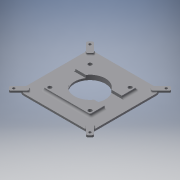
# Autodesk Inventor part: LX4000 Cuvette adapter
Saved by Autodesk Inventor 2016 (Build 200138000, 138)
## iProperties
Created: 2015-05-08
Part Number: LX4000 Cuvette adapter
Material: Generic
Document SubType Name: Modeling
Designer: kthorn
Density: 1 g/cm^3
Appearance: Default
Author: kthorn
Autodesk Inventor part; units mm, degrees
ref_plane "YZ Plane" through (0, 0, 0) normal (1, 0, 0) x (0, 1, 0)
ref_plane "XZ Plane" through (0, 0, 0) normal (0, 1, 0) x (-1, 0, 0)
ref_plane "XY Plane" through (0, 0, 0) normal (0, 0, 1) x (1, 0, 0)
sketch "Sketch1" plane through (0, 0, 0) normal (0, 0, 1) x (1, 0, 0)
  line L0 (-34.939227, 36.850829) -> (65.060773, 36.850829)
  line L1 (73.060773, 28.850829) -> (73.060773, -71.149171)
  line L2 (65.060773, -79.149171) -> (-34.939227, -79.149171)
  line L3 (-42.939227, -71.149171) -> (-42.939227, 28.850829)
  arc A0 (-34.939227, 36.850829) -> (-42.939227, 28.850829) centre (-34.939227, 28.850829) ccw
  arc A1 (-42.939227, -71.149171) -> (-34.939227, -79.149171) centre (-34.939227, -71.149171) ccw
  arc A2 (65.060773, -79.149171) -> (73.060773, -71.149171) centre (65.060773, -71.149171) ccw
  arc A3 (73.060773, 28.850829) -> (65.060773, 36.850829) centre (65.060773, 28.850829) ccw
  point P0 (0, 0)
  point P1 (-42.939227, 36.850829)
  point P2 (73.060773, 36.850829)
  dimension "d0" = 116
  dimension "d2" = 8
  constraints: 8 end point, 8 point on circle, 8 tangent, 4 centre point, 4 point on line, 3 equal radius, 2 parallel, 2 perpendicular, 1 horizontal
  measures "d0" distance of point (-42.939, 36.851) point (73.061, 36.851)
  measures "d2" radius of A0
extrude "Extrusion1" add sketch "Sketch1" along normal blind 3.1
sketch "Sketch3" plane through (0, 0, 3.1) normal (0, 0, 1) x (1, 0, 0)
  line L0 (-34.939227, -79.149171) -> (65.060773, -79.149171)
  line L1 (65.060773, 36.850829) -> (-34.939227, 36.850829)
  line L2 (-42.939227, -71.149171) -> (-42.939227, -79.149171) construction
  line L3 (-34.939227, -79.149171) -> (-42.939227, -79.149171) construction
  line L4 (-42.939227, -79.149171) -> (-42.939227, -82.899171) construction
  line L5 (-42.939227, -82.899171) -> (-46.689227, -82.899171) construction
  line L6 (-32.658004, -75.231909) -> (-46.093032, -88.666938)
  line L7 (-48.92146, -88.666938) -> (-52.456993, -85.131404)
  line L8 (-52.456993, -82.302977) -> (-39.021965, -68.867948)
  line L9 (-36.193538, -68.867948) -> (-32.658004, -72.403482)
  line L10 (-46.689227, -82.899171) -> (-46.689227, -86.899171) construction
  line L11 (-46.689227, -86.899171) -> (-50.689227, -86.899171) construction
  circle A0 centre (-46.689227, -82.899171) radius 2
  arc A1 (-52.456993, -82.302977) -> (-52.456993, -85.131404) centre (-51.04278, -83.71719) ccw
  arc A2 (-48.92146, -88.666938) -> (-46.093032, -88.666938) centre (-47.507246, -87.252724) ccw
  arc A3 (-36.193538, -68.867948) -> (-39.021965, -68.867948) centre (-37.607751, -70.282162) ccw
  arc A4 (-32.658004, -75.231909) -> (-32.658004, -72.403482) centre (-34.072217, -73.817696) ccw
  line L12 (-42.939227, 28.850829) -> (-42.939227, -71.149171)
  arc A5 (-42.939227, -71.149171) -> (-34.939227, -79.149171) centre (-34.939227, -71.149171) ccw
  line L13 (-34.939227, -79.149171) -> (65.060773, -79.149171)
  arc A6 (65.060773, -79.149171) -> (73.060773, -71.149171) centre (65.060773, -71.149171) ccw
  line L14 (73.060773, -71.149171) -> (73.060773, 28.850829)
  arc A7 (73.060773, 28.850829) -> (65.060773, 36.850829) centre (65.060773, 28.850829) ccw
  line L15 (65.060773, 36.850829) -> (-34.939227, 36.850829)
  arc A8 (-34.939227, 36.850829) -> (-42.939227, 28.850829) centre (-34.939227, 28.850829) ccw
  line L16 (15.060773, -79.149171) -> (15.060773, 36.850829) construction
  line L17 (73.060773, -21.149171) -> (-42.939227, -21.149171) construction
  line L18 (73.060773, -71.149171) -> (73.060773, -79.149171) construction
  line L19 (65.060773, -79.149171) -> (73.060773, -79.149171) construction
  line L20 (73.060773, -79.149171) -> (73.060773, -82.899171) construction
  line L21 (73.060773, -82.899171) -> (76.810773, -82.899171) construction
  line L22 (62.779551, -75.231909) -> (76.214579, -88.666938)
  line L23 (79.043007, -88.666938) -> (82.57854, -85.131404)
  line L24 (82.57854, -82.302977) -> (69.143512, -68.867948)
  line L25 (66.315084, -68.867948) -> (62.779551, -72.403482)
  line L26 (76.810773, -82.899171) -> (76.810773, -86.899171) construction
  line L27 (76.810773, -86.899171) -> (80.810773, -86.899171) construction
  circle A9 centre (76.810773, -82.899171) radius 2
  arc A10 (82.57854, -85.131404) -> (82.57854, -82.302977) centre (81.164327, -83.71719) ccw
  arc A11 (76.214579, -88.666938) -> (79.043007, -88.666938) centre (77.628793, -87.252724) ccw
  arc A12 (69.143512, -68.867948) -> (66.315084, -68.867948) centre (67.729298, -70.282162) ccw
  arc A13 (62.779551, -72.403482) -> (62.779551, -75.231909) centre (64.193764, -73.817696) ccw
  arc A14 (65.060773, -79.149171) -> (73.060773, -71.149171) centre (65.060773, -71.149171) ccw
  line L28 (-42.939227, 28.850829) -> (-42.939227, 36.850829) construction
  line L29 (-34.939227, 36.850829) -> (-42.939227, 36.850829) construction
  line L30 (-42.939227, 36.850829) -> (-42.939227, 40.600829) construction
  line L31 (-42.939227, 40.600829) -> (-46.689227, 40.600829) construction
  line L32 (-32.658004, 32.933567) -> (-46.093032, 46.368596)
  line L33 (-48.92146, 46.368596) -> (-52.456993, 42.833062)
  line L34 (-52.456993, 40.004635) -> (-39.021965, 26.569606)
  line L35 (-36.193538, 26.569606) -> (-32.658004, 30.10514)
  line L36 (-46.689227, 40.600829) -> (-46.689227, 44.600829) construction
  line L37 (-46.689227, 44.600829) -> (-50.689227, 44.600829) construction
  circle A15 centre (-46.689227, 40.600829) radius 2
  arc A16 (-52.456993, 42.833062) -> (-52.456993, 40.004635) centre (-51.04278, 41.418849) ccw
  arc A17 (-46.093032, 46.368596) -> (-48.92146, 46.368596) centre (-47.507246, 44.954382) ccw
  arc A18 (-39.021965, 26.569606) -> (-36.193538, 26.569606) centre (-37.607751, 27.98382) ccw
  arc A19 (-32.658004, 30.10514) -> (-32.658004, 32.933567) centre (-34.072217, 31.519354) ccw
  arc A20 (-34.939227, 36.850829) -> (-42.939227, 28.850829) centre (-34.939227, 28.850829) ccw
  arc A21 (73.060773, 28.850829) -> (65.060773, 36.850829) centre (65.060773, 28.850829) ccw
  arc A22 (62.779551, 32.933567) -> (62.779551, 30.10514) centre (64.193764, 31.519354) ccw
  line L38 (66.315084, 26.569606) -> (62.779551, 30.10514)
  arc A23 (66.315084, 26.569606) -> (69.143512, 26.569606) centre (67.729298, 27.98382) ccw
  arc A24 (73.060773, 28.850829) -> (65.060773, 36.850829) centre (65.060773, 28.850829) ccw
  line L39 (73.060773, 28.850829) -> (73.060773, 36.850829) construction
  line L40 (65.060773, 36.850829) -> (73.060773, 36.850829) construction
  line L41 (73.060773, 36.850829) -> (73.060773, 40.600829) construction
  line L42 (73.060773, 40.600829) -> (76.810773, 40.600829) construction
  line L43 (62.779551, 32.933567) -> (76.214579, 46.368596)
  line L44 (79.043007, 46.368596) -> (82.57854, 42.833062)
  line L45 (82.57854, 40.004635) -> (69.143512, 26.569606)
  line L46 (76.810773, 40.600829) -> (76.810773, 44.600829) construction
  line L47 (76.810773, 44.600829) -> (80.810773, 44.600829) construction
  circle A25 centre (76.810773, 40.600829) radius 2
  arc A26 (82.57854, 40.004635) -> (82.57854, 42.833062) centre (81.164327, 41.418849) ccw
  arc A27 (79.043007, 46.368596) -> (76.214579, 46.368596) centre (77.628793, 44.954382) ccw
  arc A28 (-42.939227, -71.149171) -> (-34.939227, -79.149171) centre (-34.939227, -71.149171) ccw
  line L48 (-34.939227, -71.149171) -> (-42.939227, -79.149171) construction
  point P0 (0, 0)
  point P1 (-31.24379, -73.817696)
  point P2 (-37.607751, -67.453734)
  point P3 (-34.425771, -70.635715)
  point P4 (61.365337, -73.817696)
  point P5 (67.729298, -67.453734)
  point P6 (64.547318, -70.635715)
  point P7 (-31.24379, 31.519354)
  point P8 (-37.607751, 25.155393)
  point P9 (-34.425771, 28.337373)
  point P10 (61.365337, 31.519354)
  point P11 (67.729298, 25.155393)
  point P12 (64.547318, 28.337373)
  dimension "d13" = 3.75
  dimension "d15" = 4
  dimension "d16" = 4
  dimension "d17" = 9
  dimension "d18" = 2
  dimension "d32" = 23
  constraints: 86 end point, 83 symmetric about line, 40 point on circle, 24 centre point, 16 point on line, 10 perpendicular, 8 tangent, 6 midpoint, 4 coincident, 3 equal radius, 2 parallel, 19 other
  measures "d13" distance of L4.end L5.end
  measures "d15" distance of L11.end L10.end
  measures "d16" diameter of A0
  measures "d17" distance of point (-37.608, -67.454) point (-31.244, -73.818)
  measures "d18" radius of A1
  measures "d32" distance between parallel lines of L7 L9
extrude "Extrusion4" add sketch "Sketch3" along normal blind 3 contours A5 L8 A3 L9 A4 L6 | L6 A2 L7 A1 L8 A5 | L22 A13 L25 A12 L24 A6 | A6 L24 A10 L23 A11 L22 | L34 A16 L33 A17 L32 A8 | A8 L32 A19 L35 A18 L34 | L45 A23 L38 A22 L43 A7 | A7 L43 A27 L44 A26 L45
fillet "Fillet1" radius 2 5 edges at (62.1938, -73.8177, 3.1) (64.5473, -70.6357, 3.1) (67.7293, -68.2822, 3.1) (71.0317, -70.7561, 3.1) (64.6677, -77.1201, 3.1)
fillet "Fillet2" radius 2 15 edges at (-32.0722, -73.8177, 3.1) (-34.4258, -70.6357, 3.1) (-37.6078, -68.2822, 3.1) (-40.9101, -70.7561, 3.1) (-34.5462, -77.1201, 3.1) (64.5473, 28.3374, 3.1) (62.1938, 31.5194, 3.1) (64.6677, 34.8217, 3.1) (71.0317, 28.4578, 3.1) (67.7293, 25.9838, 3.1) (-40.9101, 28.4578, 3.1) (-34.4258, 28.3374, 3.1) (-32.0722, 31.5194, 3.1) (-34.5462, 34.8217, 3.1) (-37.6078, 25.9838, 3.1)
sketch "Sketch5" plane through (0, 0, 3.1) normal (0, 0, 1) x (1, 0, 0)
  line L0 (-17.439227, 11.350829) -> (47.560773, 11.350829) construction
  line L1 (47.560773, 11.350829) -> (47.560773, -53.649171) construction
  line L2 (47.560773, -53.649171) -> (-17.439227, -53.649171) construction
  line L3 (-17.439227, -53.649171) -> (-17.439227, 11.350829) construction
  line L4 (-42.939227, 27.658441) -> (-40.436178, 25.155393) construction
  line L5 (-42.939227, 27.658441) -> (-42.939227, -69.956783) construction
  line L6 (-40.436178, -67.453734) -> (-42.939227, -69.956783) construction
  arc A0 (-34.779324, -67.453734) -> (-40.436178, -67.453734) centre (-37.607751, -70.282162) ccw construction
  line L7 (-31.24379, -70.989268) -> (-34.779324, -67.453734) construction
  arc A1 (-31.24379, -76.646123) -> (-31.24379, -70.989268) centre (-34.072217, -73.817696) ccw construction
  line L8 (-33.746838, -79.149171) -> (-31.24379, -76.646123) construction
  line L9 (-33.746838, -79.149171) -> (63.868385, -79.149171) construction
  line L10 (61.365337, -76.646123) -> (63.868385, -79.149171) construction
  arc A2 (61.365337, -70.989268) -> (61.365337, -76.646123) centre (64.193764, -73.817696) ccw construction
  line L11 (64.900871, -67.453734) -> (61.365337, -70.989268) construction
  arc A3 (70.557725, -67.453734) -> (64.900871, -67.453734) centre (67.729298, -70.282162) ccw construction
  line L12 (73.060773, -69.956783) -> (70.557725, -67.453734) construction
  line L13 (73.060773, -69.956783) -> (73.060773, 27.658441) construction
  line L14 (70.557725, 25.155393) -> (73.060773, 27.658441) construction
  arc A4 (64.900871, 25.155393) -> (70.557725, 25.155393) centre (67.729298, 27.98382) ccw construction
  line L15 (61.365337, 28.690926) -> (64.900871, 25.155393) construction
  arc A5 (61.365337, 34.347781) -> (61.365337, 28.690926) centre (64.193764, 31.519354) ccw construction
  line L16 (63.868385, 36.850829) -> (61.365337, 34.347781) construction
  line L17 (63.868385, 36.850829) -> (-33.746838, 36.850829) construction
  line L18 (-31.24379, 34.347781) -> (-33.746838, 36.850829) construction
  arc A6 (-31.24379, 28.690926) -> (-31.24379, 34.347781) centre (-34.072217, 31.519354) ccw construction
  line L19 (-34.779324, 25.155393) -> (-31.24379, 28.690926) construction
  arc A7 (-40.436178, 25.155393) -> (-34.779324, 25.155393) centre (-37.607751, 27.98382) ccw construction
  line L20 (15.060773, 11.350829) -> (15.060773, 36.850829) construction
  line L21 (63.868385, 36.850829) -> (-33.746838, 36.850829) construction
  line L22 (15.060773, -53.649171) -> (15.060773, -79.149171) construction
  line L23 (47.560773, -21.149171) -> (73.060773, -21.149171) construction
  line L24 (73.060773, -69.956783) -> (73.060773, 27.658441) construction
  line L25 (-17.439227, -21.149171) -> (-42.939227, -21.149171) construction
  circle A8 centre (-17.439227, 11.350829) radius 3
  circle A9 centre (47.560773, 11.350829) radius 3
  circle A10 centre (47.560773, -53.649171) radius 3
  circle A11 centre (-17.439227, -53.649171) radius 3
  line L26 (-17.439227, 11.350829) -> (47.560773, -53.649171) construction
  circle A12 centre (15.060773, -21.149171) radius 25
  point P0 (0, 0)
  dimension "d33" = 6
  dimension "d34" = 65
  dimension "d35" = 50
  constraints: 18 end point, 9 midpoint, 5 centre point, 5 perpendicular, 4 coincident, 3 equal length, 3 equal radius, 2 parallel, 1 horizontal
  measures "d33" diameter of A8
  measures "d34" distance of L0.start L0.end
  measures "d35" diameter of A12
extrude "Extrusion7" cut sketch "Sketch5" against normal through all
sketch "Sketch8" plane through (0, 0, 3.1) normal (0, 0, 1) x (1, 0, 0)
  circle A0 centre (15.060773, -21.149171) radius 25
  circle A1 centre (-17.439227, 11.350829) radius 3
  circle A2 centre (47.560773, 11.350829) radius 3
  circle A3 centre (47.560773, -53.649171) radius 3
  circle A4 centre (-17.439227, -53.649171) radius 3
  line L0 (-20.439227, 16.350829) -> (50.560773, 16.350829)
  line L1 (52.560773, 14.350829) -> (52.560773, -56.649171)
  line L2 (50.560773, -58.649171) -> (-20.439227, -58.649171)
  line L3 (-22.439227, -56.649171) -> (-22.439227, 14.350829)
  line L4 (15.060773, -21.149171) -> (52.560773, 16.350829) construction
  line L5 (15.060773, -21.149171) -> (52.560773, -58.649171) construction
  line L6 (15.060773, -21.149171) -> (-22.439227, -58.649171) construction
  arc A5 (-20.439227, 16.350829) -> (-22.439227, 14.350829) centre (-20.439227, 14.350829) ccw
  arc A6 (52.560773, 14.350829) -> (50.560773, 16.350829) centre (50.560773, 14.350829) ccw
  arc A7 (-22.439227, -56.649171) -> (-20.439227, -58.649171) centre (-20.439227, -56.649171) ccw
  arc A8 (50.560773, -58.649171) -> (52.560773, -56.649171) centre (50.560773, -56.649171) ccw
  point P0 (0, 0)
  point P1 (-22.439227, 16.350829)
  dimension "d39" = 75
  dimension "d40" = 2
  constraints: 14 end point, 8 point on circle, 8 point on line, 8 tangent, 4 centre point, 4 perpendicular, 3 equal radius, 2 parallel, 1 horizontal
  measures "d39" distance of point (-22.439, 16.351) L4.end
  measures "d40" radius of A5
extrude "Extrusion8" add sketch "Sketch8" along normal blind 4.4
fillet "Fillet3" radius 3.5 8 edges at (-21.8534, -58.0634, 3.1) (-22.4392, -21.1492, 3.1) (-21.8534, 15.765, 3.1) (15.0608, 16.3508, 3.1) (51.975, 15.765, 3.1) (52.5608, -21.1492, 3.1) (51.975, -58.0634, 3.1) (15.0608, -58.6492, 3.1)
sketch "Sketch9" plane through (0, 0, 7.5) normal (0, 0, 1) x (1, 0, 0)
  circle A0 centre (15.060773, -21.149171) radius 25
  circle A1 centre (-17.439227, -53.649171) radius 3
  circle A2 centre (47.560773, -53.649171) radius 3
  circle A3 centre (47.560773, 11.350829) radius 3
  circle A4 centre (-17.439227, 11.350829) radius 3
  line L0 (-22.439227, 14.350829) -> (-22.439227, -56.649171)
  arc A5 (-22.439227, -56.649171) -> (-20.439227, -58.649171) centre (-20.439227, -56.649171) ccw
  line L1 (-20.439227, -58.649171) -> (50.560773, -58.649171)
  arc A6 (50.560773, -58.649171) -> (52.560773, -56.649171) centre (50.560773, -56.649171) ccw
  line L2 (52.560773, -56.649171) -> (52.560773, 14.350829)
  arc A7 (52.560773, 14.350829) -> (50.560773, 16.350829) centre (50.560773, 14.350829) ccw
  line L3 (50.560773, 16.350829) -> (-20.439227, 16.350829)
  arc A8 (-20.439227, 16.350829) -> (-22.439227, 14.350829) centre (-20.439227, 14.350829) ccw
  line L4 (-42.939227, -7.149171) -> (-42.939227, -35.149171)
  line L5 (-42.939227, -7.149171) -> (-5.651542, -7.149171)
  line L6 (-42.939227, -35.149171) -> (-5.651542, -35.149171)
  line L7 (-20.439227, 16.350829) -> (50.560773, 16.350829) construction
  line L8 (15.060773, 16.350829) -> (15.060773, -58.649171) construction
  line L9 (-20.439227, -58.649171) -> (50.560773, -58.649171) construction
  line L10 (-42.939227, 27.658441) -> (-40.436178, 25.155393)
  line L11 (-42.939227, 27.658441) -> (-42.939227, -69.956783)
  line L12 (-40.436178, -67.453734) -> (-42.939227, -69.956783)
  arc A9 (-34.779324, -67.453734) -> (-40.436178, -67.453734) centre (-37.607751, -70.282162) ccw
  line L13 (-31.24379, -70.989268) -> (-34.779324, -67.453734)
  arc A10 (-31.24379, -76.646123) -> (-31.24379, -70.989268) centre (-34.072217, -73.817696) ccw
  line L14 (-33.746838, -79.149171) -> (-31.24379, -76.646123)
  line L15 (-33.746838, -79.149171) -> (63.868385, -79.149171)
  line L16 (61.365337, -76.646123) -> (63.868385, -79.149171)
  arc A11 (61.365337, -70.989268) -> (61.365337, -76.646123) centre (64.193764, -73.817696) ccw
  line L17 (64.900871, -67.453734) -> (61.365337, -70.989268)
  arc A12 (70.557725, -67.453734) -> (64.900871, -67.453734) centre (67.729298, -70.282162) ccw
  line L18 (73.060773, -69.956783) -> (70.557725, -67.453734)
  line L19 (73.060773, -69.956783) -> (73.060773, 27.658441)
  line L20 (70.557725, 25.155393) -> (73.060773, 27.658441)
  arc A13 (64.900871, 25.155393) -> (70.557725, 25.155393) centre (67.729298, 27.98382) ccw
  line L21 (61.365337, 28.690926) -> (64.900871, 25.155393)
  arc A14 (61.365337, 34.347781) -> (61.365337, 28.690926) centre (64.193764, 31.519354) ccw
  line L22 (63.868385, 36.850829) -> (61.365337, 34.347781)
  line L23 (63.868385, 36.850829) -> (-33.746838, 36.850829)
  line L24 (-31.24379, 34.347781) -> (-33.746838, 36.850829)
  arc A15 (-31.24379, 28.690926) -> (-31.24379, 34.347781) centre (-34.072217, 31.519354) ccw
  line L25 (-34.779324, 25.155393) -> (-31.24379, 28.690926)
  arc A16 (-40.436178, 25.155393) -> (-34.779324, 25.155393) centre (-37.607751, 27.98382) ccw
  arc A17 (-25.939227, -56.649171) -> (-20.439227, -62.149171) centre (-20.439227, -56.649171) ccw
  line L26 (-25.939227, 14.350829) -> (-25.939227, -56.649171)
  arc A18 (-20.439227, 19.850829) -> (-25.939227, 14.350829) centre (-20.439227, 14.350829) ccw
  line L27 (50.560773, 19.850829) -> (-20.439227, 19.850829)
  arc A19 (56.060773, 14.350829) -> (50.560773, 19.850829) centre (50.560773, 14.350829) ccw
  line L28 (56.060773, -56.649171) -> (56.060773, 14.350829)
  arc A20 (50.560773, -62.149171) -> (56.060773, -56.649171) centre (50.560773, -56.649171) ccw
  line L29 (-20.439227, -62.149171) -> (50.560773, -62.149171)
  arc A21 (-5.651542, -7.149171) -> (-5.651542, -35.149171) centre (15.060773, -21.149171) ccw
  line L30 (73.060773, -7.149171) -> (73.060773, -35.149171)
  line L31 (73.060773, -7.149171) -> (35.773089, -7.149171)
  line L32 (73.060773, -35.149171) -> (35.773089, -35.149171)
  arc A22 (35.773089, -35.149171) -> (35.773089, -7.149171) centre (15.060773, -21.149171) ccw
  point P0 (0, 0)
  point P1 (-42.939227, -21.149171)
  point P2 (73.060773, -21.149171)
  dimension "d44" = 28
  constraints: 14 end point, 6 point on circle, 5 symmetric about line, 4 midpoint, 2 centre point, 1 horizontal, 1 parallel, 1 vertical, 1 other
  measures "d44" distance of L4.start L4.end
extrude "Extrusion9" cut sketch "Sketch9" against normal up to surface (4.4 mm away) contours A0 L31 L2 L32 | A0 L6 L0 L5 | L31 L28 L32 L2 | L0 L6 L26 L5 | L31 L19 L32 L28 | L26 L6 L4 L5
body "Solid1"
